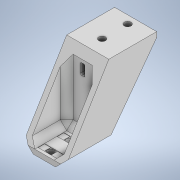
# Autodesk Inventor part: Soporte Actuador
Saved by Autodesk Inventor 2020.3 (Build 243373000, 373)
## iProperties
Created: 2021-02-18
Part Number: Soporte Actuador
Material: Generic
Document SubType Name: Modeling
Designer: juanp
Density: 1 g/cm^3
Appearance: Default
Author: juanp
Autodesk Inventor part; units mm, degrees
ref_plane "YZ Plane" through (0, 0, 0) normal (1, 0, 0) x (0, 1, 0)
ref_plane "XZ Plane" through (0, 0, 0) normal (0, 1, 0) x (-1, 0, 0)
ref_plane "XY Plane" through (0, 0, 0) normal (0, 0, 1) x (1, 0, 0)
sketch "Sketch7" plane through (0, 0, 0) normal (1, 0, 0) x (0, 1, 0)
  line L0 (0, 0) -> (4, 0)
  line L1 (4, 0) -> (4, -30)
  line L2 (4, -30) -> (0, -30)
  line L3 (0, -30) -> (0, 0)
  line L4 (60, -34) -> (56, -34)
  line L5 (56, -34) -> (56, -71.5)
  line L6 (56, -71.5) -> (60, -71.5)
  line L7 (60, -71.5) -> (60, -34)
  line L8 (4, 0) -> (60, -34)
  line L9 (0, -30) -> (56, -71.5)
  line L10 (56, -34) -> (5.3976, -34)
  line L11 (53.4118, -30) -> (4, -30)
  dimension "d22" = 4
  dimension "d24" = 60
  dimension "d25" = 4
  dimension "d30" = 30
  dimension "d34" = 37.5
  constraints: 24 end point, 6 parallel, 3 horizontal, 2 perpendicular, 2 point on line
  measures "d22" distance of L5.end L6.end
  measures "d24" distance between parallel lines of L7 L3
  measures "d25" distance between parallel lines of L10 L11
  measures "d30" distance between parallel lines of L2 L0
  measures "d34" distance between parallel lines of L6 L4
extrude "Extrusion8" add sketch "Sketch7" along normal mid plane 25 contours L0 L1 L2 L3 | L2 L11 L8 L4 L10 L9 | L7 L6 L5 L4
sketch "Sketch8" plane through (12.5, 0, 0) normal (1, 0, 0) x (0, 0, -1)
  line L0 (0, 4) -> (34, 60) projected
  line L1 (30, 53.4118) -> (30, 4) projected
  line L2 (30, 4) -> (0, 4) projected
  line L3 (0, 0) -> (30, 0) projected
  line L4 (0, 4) -> (0, 0) projected
  line L5 (30, 0) -> (34, 5.3976) projected
  line L6 (34, 5.3976) -> (34, 56) projected
  line L7 (34, 56) -> (71.5, 56) projected
  line L8 (71.5, 60) -> (34, 60) projected
  line L9 (71.5, 56) -> (71.5, 60) projected
  line L10 (30, 0) -> (71.5, 56) projected
extrude "Extrusion9" add sketch "Sketch8" along normal blind 4
mirror "Mirror2" about plane through (0, 0, 0) normal (1, 0, 0) of "Extrusion9"
chamfer "Chamfer1" distance 5 angle 45 10 edges at (12.5, 30.6988, -34) (0, 56, -34) (12.5, 56, -52.75) (-12.5, 56, -52.75) (-12.5, 30.6988, -34) (0, 4, -30) (-12.5, 4, -15) (-12.5, 28.7059, -30) (12.5, 28.7059, -30) (12.5, 4, -15)
sketch "Sketch9" plane through (-7.5, 4, 0) normal (0, 1, 0) x (1, 0, 0)
  line L0 (7.5, 0) -> (7.5, 5) construction
  line L1 (7.5, 5) -> (7.5, 20) construction
  circle A0 centre (7.5, 20) radius 2.65
  circle A1 centre (7.5, 5) radius 2.65
  circle A2 centre (7.5, 5) radius 4.25 construction
  circle A3 centre (7.5, 20) radius 4.25 construction
  dimension "d35" = 5
  dimension "d36" = 15
  dimension "d37" = 5.3
  dimension "d38" = 5.3
  dimension "d43" = 8.5
  dimension "d44" = 8.5
  constraints: 4 centre point, 4 coincident, 4 end point, 1 point on line, 1 vertical
  measures "d35" distance of L0.start L0.end
  measures "d36" distance of L0.end L1.end
  measures "d37" diameter of A0
  measures "d38" diameter of A1
  measures "d43" diameter of A2
  measures "d44" diameter of A3
sketch "Sketch10" plane through (-7.5, 56, -39) normal (0, -1, 0) x (1, 0, 0)
  line L0 (0, 0) -> (15, 0) projected
  line L1 (7.5, 0) -> (7.5, -6.25) construction
  line L2 (7.5, -6.25) -> (7.5, -26.25) construction
  line L3 (7.5, -26.25) -> (7.5, -32.5) construction
  line L4 (-9, -32.5) -> (24, -32.5) projected
  circle A0 centre (7.5, -6.25) radius 2.65
  circle A1 centre (7.5, -26.25) radius 2.65
  circle A2 centre (7.5, -6.25) radius 4.75 construction
  circle A3 centre (7.5, -26.25) radius 4.75 construction
  point P0 (7.5, 39)
  dimension "d39" = 20
  dimension "d40" = 5.3
  dimension "d41" = 9.5
  dimension "d42" = 9.5
  constraints: 6 end point, 4 centre point, 4 coincident, 2 midpoint, 1 collinear, 1 equal radius, 1 point on line, 1 vertical
  measures "d39" distance of L1.end L2.end
  measures "d40" diameter of A0
  measures "d41" diameter of A2
  measures "d42" diameter of A3
extrude "Extrusion10" cut sketch "Sketch9" against normal through all both and the other way through all
extrude "Extrusion11" cut sketch "Sketch10" along normal through all both and the other way through all
chamfer "Chamfer3" distance 7.75 angle 45 2 edges at (-16.5, 0, -15) (16.5, 0, -15)
sketch "Sketch12" plane through (-7.5, 4, 0) normal (0, 1, 0) x (1, 0, 0)
  circle A0 centre (7.5, 20) radius 2.65 projected
  circle A1 centre (7.5, 5) radius 2.65 projected
  line L0 (0, 0) -> (0, 25) projected
  line L1 (0, 0) -> (15, 0) projected
  line L2 (15, 25) -> (15, 0) projected
  line L3 (0, 25) -> (15, 25) projected
  line L4 (15, 22.65) -> (0, 22.65)
  line L5 (0, 17.35) -> (15, 17.35)
  line L6 (0, 7.65) -> (15, 7.65)
  line L7 (0, 2.35) -> (15, 2.35)
  line L8 (4.85, 17.35) -> (10.15, 17.35)
  line L9 (10.15, 17.35) -> (10.15, 22.65)
  line L10 (10.15, 22.65) -> (4.85, 22.65)
  line L11 (4.85, 22.65) -> (4.85, 17.35)
  line L12 (4.85, 17.35) -> (10.15, 22.65) construction
  line L13 (10.15, 17.35) -> (4.85, 22.65) construction
  line L14 (4.85, 2.35) -> (10.15, 2.35)
  line L15 (10.15, 2.35) -> (10.15, 7.65)
  line L16 (10.15, 7.65) -> (4.85, 7.65)
  line L17 (4.85, 7.65) -> (4.85, 2.35)
  line L18 (4.85, 2.35) -> (10.15, 7.65) construction
  line L19 (10.15, 2.35) -> (4.85, 7.65) construction
  point P0 (7.5, 0)
  point P1 (7.5, 2.35)
  point P2 (7.5, 7.65)
  point P3 (7.5, 22.65)
  point P4 (7.5, 17.35)
  point P5 (4.85, 7.65)
  point P6 (4.85, 5)
  point P7 (10.15, 2.35)
  point P8 (10.15, 5)
  point P9 (4.85, 2.35)
  point P10 (4.85, 20)
  point P11 (10.15, 20)
  constraints: 32 end point, 11 point on line, 6 perpendicular, 5 tangent, 4 midpoint, 4 parallel, 2 horizontal
extrude "Extrusion13" cut sketch "Sketch12" against normal blind 0.3 contours L9 L5 A0 | L9 L4 L2 L5 | A0 L4 L9 | A0 L11 L4 | L5 L11 A0 | L11 L5 L0 L4 | L2 L7 L15 L6 | L6 L17 L7 L0 | L15 A1 L6 | L6 A1 L17 | L7 A1 L15 | L17 A1 L7
extrude "Extrusion14" cut sketch "Sketch12" against normal blind 0.6 contours L9 L5 A0 | A0 L4 L9 | A0 L11 L4 | L5 L11 A0 | L15 A1 L6 | L6 A1 L17 | L7 A1 L15 | L17 A1 L7
sketch "Sketch13" plane through (7.5, 5.3976, -34) normal (0, 0, -1) x (-1, 0, 0)
  line L0 (9, 37.3095) -> (6, 37.3095) construction
  line L1 (6, 37.3095) -> (6, 45.3095) construction
  line L2 (6, 45.3095) -> (9, 45.3095) construction
  line L3 (9, 45.3095) -> (9, 37.3095) construction
  line L4 (9.2929, 44.6024) -> (9.2929, 38.0166)
  line L5 (8.2929, 37.0166) -> (6.7071, 37.0166)
  line L6 (5.7071, 38.0166) -> (5.7071, 44.6024)
  line L7 (8.2929, 45.6024) -> (6.7071, 45.6024)
  arc A0 (9.2929, 44.6024) -> (8.2929, 45.6024) centre (8.2929, 44.6024) ccw
  arc A1 (8.2929, 37.0166) -> (9.2929, 38.0166) centre (8.2929, 38.0166) ccw
  arc A2 (5.7071, 38.0166) -> (6.7071, 37.0166) centre (6.7071, 38.0166) ccw
  arc A3 (6.7071, 45.6024) -> (5.7071, 44.6024) centre (6.7071, 44.6024) ccw
  line L8 (0, 45.6024) -> (15, 45.6024) projected
  point P0 (7.5, -5.3976)
  point P1 (7.5, 45.6024)
  dimension "d64" = 8
  dimension "d65" = 3
  dimension "d66" = 1
  constraints: 16 end point, 12 point on circle, 8 tangent, 4 centre point, 3 equal radius, 3 horizontal, 2 midpoint, 2 parallel, 2 vertical, 1 perpendicular
  measures "d64" distance of L1.end L0.end
  measures "d65" distance of L0.start L0.end
  measures "d66" radius of A2
extrude "Extrusion15" cut sketch "Sketch13" against normal through all
body "Solid2"
